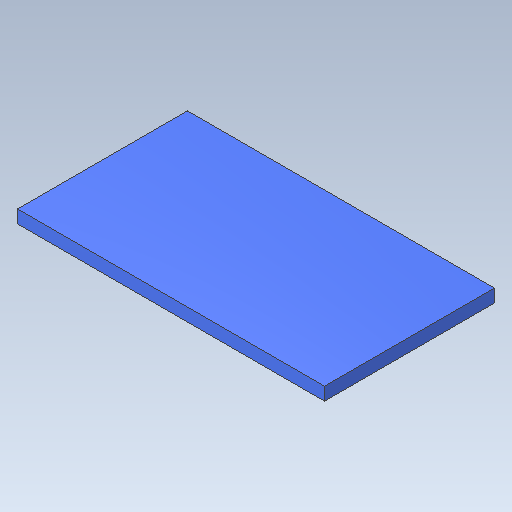
# Autodesk Inventor part: Lipo Charger Circuit
Saved by Autodesk Inventor 2020 (Build 240168000, 168)
## iProperties
Created: 2019-01-12
Part Number: Lipo Charger Circuit
Material: Generic
Document SubType Name: Modeling
Designer: LSabe
Density: 1 g/cm^3
Appearance: Default
Author: LSabe
Autodesk Inventor part; units mm, degrees
ref_plane "YZ Plane" through (0, 0, 0) normal (1, 0, 0) x (0, 1, 0)
ref_plane "XZ Plane" through (0, 0, 0) normal (0, 1, 0) x (-1, 0, 0)
sketch "Sketch1" plane through (0, 0, 0) normal (0, 1, 0) x (-1, 0, 0)
  line L0 (0, 0) -> (-90.17, 0)
  line L1 (-90.17, 0) -> (-90.17, -49.911)
  line L2 (-90.17, -49.911) -> (0, -49.911)
  line L3 (0, -49.911) -> (0, 0)
  dimension "d0" = 90.17
  dimension "d1" = 49.911
  constraints: 8 end point, 2 parallel, 1 horizontal, 1 perpendicular
  measures "d0" distance of L2.end L1.end
  measures "d1" distance of L1.end L0.end
extrude "Extrusion1" add sketch "Sketch1" along normal blind 3.81
ref_plane "Midplane" through (45.085, 0, 0) normal (1, 0, 0) x (0, 0, -1)
body "Solid1"
